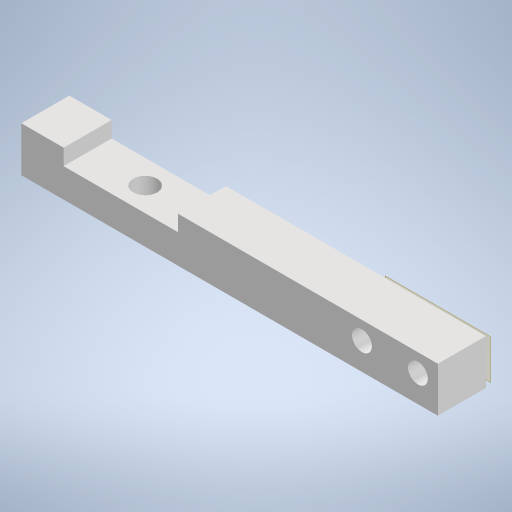
# Autodesk Inventor part: крепеж тсрт
Saved by Autodesk Inventor 2024.2 (Build 282272000, 272)
## iProperties
Created: 2026-03-12
Part Number: крепеж тсрт
Material: Типовые
Document SubType Name: Modeling
Designer: Service
Density: 1 g/cm^3
Appearance: По умолчанию
Author: Service
Autodesk Inventor part; units mm, degrees
ref_plane "YZ Plane" through (0, 0, 0) normal (1, 0, 0) x (0, 1, 0)
ref_plane "XZ Plane" through (0, 0, 0) normal (0, 1, 0) x (-1, 0, 0)
ref_plane "XY Plane" through (0, 0, 0) normal (0, 0, 1) x (1, 0, 0)
ref_plane "РабПлоскость1" through (8.6347, 23.8825, 435.6127) normal (0, 0, 1) x (0, -1, 0)
sketch "Эскиз1" plane through (8.6347, 23.8825, 435.6127) normal (0, 0, 1) x (0, -1, 0)
  line L0 (11.5, 6) -> (11.5, -6) projected
  line L1 (15, -6) -> (11.5, -6) projected
  arc A0 (15, -6) -> (16, -5) centre (15, -5) ccw projected
  line L2 (16, -1.25) -> (16, -5) projected
  line L3 (14, -1.25) -> (16, -1.25) projected
  arc A1 (12.8, -0.05) -> (14, -1.25) centre (14, -0.05) ccw projected
  line L4 (12.8, 0.05) -> (12.8, -0.05) projected
  arc A2 (14, 1.25) -> (12.8, 0.05) centre (14, 0.05) ccw projected
  line L5 (16, 1.25) -> (14, 1.25) projected
  line L6 (16, 5) -> (16, 1.25) projected
  arc A3 (16, 5) -> (15, 6) centre (15, 5) ccw projected
  line L7 (11.5, 6) -> (15, 6) projected
  circle A4 centre (13.75, 3.5) radius 1.25 projected
  circle A5 centre (13.75, -3.5) radius 1.25 projected
  line L8 (11.5, 6) -> (17.129, 6)
  line L9 (17.129, 6) -> (17.129, -46.099)
  line L10 (17.129, -46.099) -> (11.5, -46.099)
  line L11 (11.5, -46.099) -> (11.5, 6)
  point P0 (23.8825, -8.6347)
  point P1 (15, 6)
  constraints: 8 end point, 2 parallel, 1 horizontal, 1 perpendicular
extrude "Выдавливание1" add sketch "Эскиз1" along normal blind 6
sketch "Эскиз2" plane through (-37.4643, 12.3825, 435.6127) normal (0, 1, 0) x (1, 0, 0)
  circle A0 centre (12.4913, -3) radius 1.5
  line L0 (52.099, -6) -> (0, -6) projected
  line L1 (0, 0) -> (52.099, 0) projected
  line L2 (5.2913, 0) -> (19.5913, 0)
  line L3 (19.5913, 0) -> (19.5913, -6)
  line L4 (19.5913, -6) -> (5.2913, -6)
  line L5 (5.2913, -6) -> (5.2913, 0)
  point P0 (37.4643, 435.6127)
  point P1 (5.2913, -3)
  point P2 (19.5913, 0)
  dimension "d2" = 3
  dimension "d3" = 3
  dimension "d4" = 7.2
  dimension "d5" = 7.1
  constraints: 8 end point, 2 parallel, 2 point on line, 1 centre point, 1 horizontal, 1 midpoint, 1 perpendicular
  measures "d2" diameter of A0
  measures "d3" distance from line of L0 A0.centre
  measures "d4" distance of point (5.291, -3) A0.centre
  measures "d5" distance from line of L3 A0.centre
extrude "Выдавливание2" cut sketch "Эскиз2" against normal blind 2
extrude "Выдавливание3" cut sketch "Эскиз2" against normal through all contours A0
